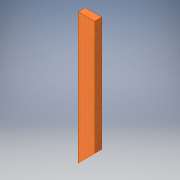
# Autodesk Inventor part: Front Face Upper Support for Slats
Saved by Autodesk Inventor 2016 (Build 200138000, 138)
## iProperties
Created: 2015-07-06
Part Number: Front Face Upper Support for Slats
Material: Wood (Cherry)
Document SubType Name: Modeling
Designer: steele
Density: 0.63 g/cm^3
Appearance: Cherry - Natural Low Gloss
Author: steele
Autodesk Inventor part; units mm, degrees
ref_plane "YZ Plane" through (0, 0, 0) normal (1, 0, 0) x (0, 1, 0)
ref_plane "XZ Plane" through (0, 0, 0) normal (0, 1, 0) x (-1, 0, 0)
ref_plane "XY Plane" through (0, 0, 0) normal (0, 0, 1) x (1, 0, 0)
sketch "Sketch3" plane through (0, 0, 0) normal (0, 0, 1) x (1, 0, 0)
  line L0 (44.45, -264.9728) -> (44.45, 353.8728)
  line L1 (44.45, 353.8728) -> (-44.45, 353.8728)
  line L2 (-44.45, 353.8728) -> (-44.45, -353.8728)
  line L3 (-44.45, -353.8728) -> (44.45, 353.8728) construction
  line L4 (44.45, -353.8728) -> (-44.45, 353.8728) construction
  line L5 (-44.45, -353.8728) -> (44.45, -264.9728)
  line L6 (44.45, -353.8728) -> (81.2736, -353.8728) construction
  point P0 (0, 0)
  dimension "d16" = 45
  dimension "d17" = 707.7456
  dimension "d18" = 88.9
  constraints: 14 end point, 2 midpoint, 1 horizontal, 1 parallel
  measures "d16" angle of L2 L5
  measures "d17" distance of L1.end L2.end
  measures "d18" distance of L0.end L1.end
extrude "Extrusion2" add sketch "Sketch3" along normal mid plane 38.1
body "Solid2"
